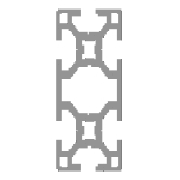
# Autodesk Inventor part: TRANSVERSAL (30X60)
Saved by Autodesk Inventor 2017 (Build 210142000, 142)
## iProperties
_CCFamilyDisplayName: 30-3060
_FrameMemberDoc: Frame Member File
_Version: 15.0.0
_GetPNFromCC: 1
Created: 2018-05-17
Part Number: TRANSVERSAL (30X60)
Material: Generic
Document SubType Name: Modeling
Standard: 8020 Metric
Designer: Luiz Gustavo
Manufacturer: 8020
Standards Organization: 8020 Metric
Language: en-US
Size Designation: 30-3060
Categories: <MemberInstance><Categories><Category DisplayName="Structural Shapes" InternalName="089c4875-fa83-4c05-b084-43b9cc11f5ed" Mnemonic="GRDR"><CategoryParameter DisplayName="Mass per Length Unit" InternalName="0bb95a10-148f-4027-a459-38d7b056702a" Mnemonic="shpmass"/><CategoryParameter DisplayName="Section Area" InternalName="1ff91680-64b0-4202-b9a3-7fd3f94bba3b" Mnemonic="secarea"/><CategoryParameter DisplayName="Radius of Gyration (x)" InternalName="25778675-03e9-40c1-b6a8-4a9ed693320d" Mnemonic="gyrradx"/><CategoryParameter DisplayName="Torsional Rigidity Modulus" InternalName="26c1ec35-5026-4c63-ad0a-751cf684a536" Mnemonic="torrigmod"/><CategoryParameter DisplayName="Distance of the Center of Gravity X-X" InternalName="26c9bdb8-9c79-4b4f-a92e-8e197583c9c4" Mnemonic="grcendistX"/><CategoryParameter DisplayName="Legacy Member ID" InternalName="340afe4f-75d7-48d3-ab7d-943f3c3da468" Mnemonic="LegacyMemberID"/><CategoryParameter DisplayName="Base Length" InternalName="42e34263-8f20-4d0e-ad48-bf1385b87c24" Mnemonic="shplen"/><CategoryParameter DisplayName="Moment of Inertia (y)" InternalName="4b9f58ea-bced-460e-81ea-3d29ca5a49e3" Mnemonic="inermomy"/><CategoryParameter DisplayName="Moment of Inertia (x)" InternalName="4cd780bc-73d7-43ac-917a-579e5cbd684d" Mnemonic="inermomx"/><CategoryParameter DisplayName="Custom Base Point" InternalName="4f1d1b73-316d-484b-a3df-9cbabb16eb77" Mnemonic="shpBasePoint"/><CategoryParameter DisplayName="Shape Height" InternalName="50274e7d-5ac0-4796-92cb-c59e54983c67" Mnemonic="shpheig"/><CategoryParameter DisplayName="Section Module (y)" InternalName="59eaa5e9-d227-48dc-b6c1-6920f96e0f95" Mnemonic="secmody"/><CategoryParameter DisplayName="Section Designation" InternalName="5a64d034-428d-49c8-ba32-7619764de20f" Mnemonic="shpdes"/><CategoryParameter DisplayName="Section Module (x)" InternalName="72cfad18-cf51-4ed4-aaa7-c6b224f8419f" Mnemonic="secmodx"/><CategoryParameter DisplayName="Torsional Section Modulus" InternalName="7c55a8dc-8844-49f9-a867-cc677b30ec9a" Mnemonic="torsecmod"/><CategoryParameter DisplayName="Shape Width" InternalName="7c717d54-a18f-4666-b4d4-573cce22c62c" Mnemonic="shpwdth"/><CategoryParameter DisplayName="Second Shape Thickness" InternalName="9251a8e1-85fd-4e47-af99-afdb762317d9" Mnemonic="shpthick2"/><CategoryParameter DisplayName="FG Authored" InternalName="9c666724-f362-4ea7-ac62-f6a007de5c69" Mnemonic="shpFGAuto"/><CategoryParameter DisplayName="Distance of the Center of Gravity Y-Y" InternalName="bcc4fb17-7af4-436a-8f8c-d0aa3b0248c5" Mnemonic="grcendistY"/><CategoryParameter DisplayName="Radius of Gyration (y)" InternalName="bfa18ebe-1636-4dbe-8d42-b263e0b73184" Mnemonic="gyrrady"/><CategoryParameter DisplayName="Shape Thickness" InternalName="d109cf76-8eb4-42fc-9800-4409734adc67" Mnemonic="shpthick"/><CategoryParameter DisplayName="Coefficient of Shear Displacement" InternalName="de4c90c6-aaa8-468f-a335-6737b311b5d3" Mnemonic="shdispc"/><Category DisplayName="Other" InternalName="f02205ff-2390-476f-921c-0b3185f88e84" Mnemonic="OTHSHP"><CategoryParameter DisplayName="Moment of Inertia (y)" InternalName="044c654e-f649-48ac-84cc-650a29ae31ca" Mnemonic="inermomy"/><CategoryParameter DisplayName="Shape Thickness" InternalName="12b1a788-9233-48fd-a933-2df8ff42b15f" Mnemonic="shpthick"/><CategoryParameter DisplayName="Mass per Length Unit" InternalName="2fd289d6-9394-4d2d-97e6-6659d7d4551d" Mnemonic="shpmass"/><CategoryParameter DisplayName="Radius of Gyration (y)" InternalName="743e1dfe-1bba-408b-b985-cf752b207386" Mnemonic="gyrrady"/><CategoryParameter DisplayName="Section Module (y)" InternalName="88b8bff9-a616-4028-93d5-ed4f79680d13" Mnemonic="secmody"/><CategoryParameter DisplayName="Section Area" InternalName="c46ecdf8-b6eb-4db9-8b25-30258930c1e3" Mnemonic="secarea"/><CategoryParameter DisplayName="Section Module (x)" InternalName="cac70804-9d39-43bb-be17-56ea1f39a6c2" Mnemonic="secmodx"/><CategoryParameter DisplayName="Moment of Inertia (x)" InternalName="ec6737bc-264f-43ed-b0bd-f6d410c2718d" Mnemonic="inermomx"/><CategoryParameter DisplayName="Radius of Gyration (x)" InternalName="ee72c61e-565e-4fd6-b448-66e1e1abcb7e" Mnemonic="gyrradx"/><Category DisplayName="8020" InternalName="79851eee-1260-43d5-80eb-d25638456875" Mnemonic="8020"/></Category></Category><Category DisplayName="DataType" InternalName="23b78d0f-2648-40c6-8793-ca6db495c9e8" Mnemonic="DATATYPE"><CategoryParameter DisplayName="DisplayName" InternalName="05415f3d-3907-474b-a020-eb9d644f4cf3" Mnemonic="DISPLAYNAME"/><CategoryParameter DisplayName="Standard" InternalName="0c0a119c-1e12-4c84-803f-101930972f5e" Mnemonic="STANDARD"/><CategoryParameter DisplayName="Description" InternalName="13903e3d-64b1-4950-80da-f627842ea37f" Mnemonic="DESCRIPTION"/><CategoryParameter DisplayName="Designation" InternalName="2675968c-4ce5-49e0-a4f5-552d29089031" Mnemonic="DESIGNATION"/><CategoryParameter DisplayName="Default Row" InternalName="2af9ec52-faaa-4026-b378-f9fa4afca842" Mnemonic="DEFAULTROW"/><CategoryParameter DisplayName="Folder Name" InternalName="3f06958e-8713-4116-9be7-ed6184ecc97b" Mnemonic="FOLDERNAME"/><CategoryParameter DisplayName="Revision Guid" InternalName="45a75005-10b1-4dfc-8d6d-dfe629f0b93c" Mnemonic="REVISIONGUID"/><CategoryParameter DisplayName="FileName" InternalName="8b46a4cc-9585-4fed-90c3-899f57e09a73" Mnemonic="FILENAME"/><CategoryParameter DisplayName="StdsOrg" InternalName="8f5914e1-4693-403f-8ab5-d37768198c9d" Mnemonic="STDSORG"/><CategoryParameter DisplayName="Family Version" InternalName="914462f6-6e19-4b14-ba84-155b9680b1d0" Mnemonic="FAMILYREVISION"/><CategoryParameter DisplayName="Standard Revision" InternalName="91d5a463-65c2-4fde-b823-3b7fea5e8e17" Mnemonic="STANDARDREVISION"/><CategoryParameter DisplayName="Member Revision" InternalName="a65d44b9-392f-4f4f-857b-e4b3d54996fe" Mnemonic="MEMBERREVISION"/><CategoryParameter DisplayName="ClipFormat" InternalName="bc51e27b-3422-4e78-93ef-cec197ddf230" Mnemonic="CLIPFORMAT"/><CategoryParameter DisplayName="Manufacturer" InternalName="cd6c7a72-a28a-4e50-99a9-2c7f4e13e5ad" Mnemonic="MANUFACTURER"/><CategoryParameter DisplayName="InternalName" InternalName="cf1d0246-76d9-4b4a-8305-fa0409afb5c1" Mnemonic="INTERNALNAME"/><CategoryParameter DisplayName="IsMetric" InternalName="e2385c5b-1ea4-4823-96a8-8de651266ec3" Mnemonic="ISMETRIC"/><Category DisplayName="Part" InternalName="c0e0b642-3bcb-4cc8-9e80-f96d35c4afa4" Mnemonic="PART"><CategoryParameter DisplayName="Part Number" InternalName="016b6077-bfbe-49bd-92c9-d8d59c39c941" Mnemonic="PARTNUMBER"/><CategoryParameter DisplayName="Stock Number" InternalName="4dba7c1c-e26c-444e-836c-b08b433409a8" Mnemonic="STOCKNUMBER"/><CategoryParameter DisplayName="Material Key" InternalName="5c9a8adb-dd2b-4535-b97f-0a94a95fe41f" Mnemonic="MATERIALKEY"/><CategoryParameter DisplayName="Material" InternalName="818a152a-d3c3-49ca-80ee-df7d91421b8e" Mnemonic="MATERIAL"/></Category></Category></Categories><FamilyTemplate Id="30-3060"><FamilyTemplateParameters><FamilyTemplateParameter ObjectType="kModelParameterObject" ValueType="xs:double" Id="12" ObjectReferenceKey="Length"/><FamilyTemplateParameter ObjectType="kPartComponentDefinitionObject" ValueType="xs:string" Id="23" SubObjectId="Material"/><FamilyTemplateParameter ObjectType="kPropertyObject" ValueType="xs:string" Id="26" ObjectReferenceKey="{32853F0F-3444-11d1-9E93-0060B03C1CA6}" SubObjectId="5"/><FamilyTemplateParameter ObjectType="kPropertyObject" ValueType="xs:string" Id="27" ObjectReferenceKey="{32853F0F-3444-11d1-9E93-0060B03C1CA6}" SubObjectId="52"/></FamilyTemplateParameters></FamilyTemplate><CategoryParameterMap><ParamToTemplateMap><ParamToTemplate CategoryParameter="//CategoryParameter[@InternalName='cf1d0246-76d9-4b4a-8305-fa0409afb5c1']" ConstantValue="ebd6c703-6585-4f80-969f-cab21f52a046"/><ParamToTemplate CategoryParameter="//CategoryParameter[@InternalName='45a75005-10b1-4dfc-8d6d-dfe629f0b93c']" ConstantValue="e073d83d-0598-4edb-9b1a-a79ba5c041d1"/><ParamToTemplate CategoryParameter="//CategoryParameter[@InternalName='3f06958e-8713-4116-9be7-ed6184ecc97b']" ConstantValue="30-3060"/><ParamToTemplate CategoryParameter="//CategoryParameter[@InternalName='8f5914e1-4693-403f-8ab5-d37768198c9d']" ConstantValue="8020 Metric"/><ParamToTemplate CategoryParameter="//CategoryParameter[@InternalName='0c0a119c-1e12-4c84-803f-101930972f5e']" TemplateParameter="18"/><ParamToTemplate CategoryParameter="//CategoryParameter[@InternalName='91d5a463-65c2-4fde-b823-3b7fea5e8e17']" TemplateParameter="19"/><ParamToTemplate CategoryParameter="//CategoryParameter[@InternalName='cd6c7a72-a28a-4e50-99a9-2c7f4e13e5ad']" ConstantValue="8020"/><ParamToTemplate CategoryParameter="//CategoryParameter[@InternalName='13903e3d-64b1-4950-80da-f627842ea37f']" TemplateParameter="22"/><ParamToTemplate CategoryParameter="//CategoryParameter[@InternalName='05415f3d-3907-474b-a020-eb9d644f4cf3']" ConstantValue="30-3060"/><ParamToTemplate CategoryParameter="//CategoryParameter[@InternalName='914462f6-6e19-4b14-ba84-155b9680b1d0']" ConstantValue="11"/><ParamToTemplate CategoryParameter="//CategoryParameter[@InternalName='bc51e27b-3422-4e78-93ef-cec197ddf230']" ConstantValue="CF_INVENTOR.STDPARTS"/><ParamToTemplate CategoryParameter="//CategoryParameter[@InternalName='e2385c5b-1ea4-4823-96a8-8de651266ec3']" ConstantValue="false"/><ParamToTemplate CategoryParameter="//CategoryParameter[@InternalName='2af9ec52-faaa-4026-b378-f9fa4afca842']" ConstantValue="1"/><ParamToTemplate CategoryParameter="//CategoryParameter[@InternalName='4f1d1b73-316d-484b-a3df-9cbabb16eb77']" ConstantValue="1"/><ParamToTemplate CategoryParameter="//CategoryParameter[@InternalName='9c666724-f362-4ea7-ac62-f6a007de5c69']" ConstantValue="1"/><ParamToTemplate CategoryParameter="//CategoryParameter[@InternalName='8b46a4cc-9585-4fed-90c3-899f57e09a73']" ConstantValue="30-3060"/><ParamToTemplate CategoryParameter="//CategoryParameter[@InternalName='a65d44b9-392f-4f4f-857b-e4b3d54996fe']" ConstantValue="3621f859-3cd7-4c8d-9d7e-184ee6a29b8c"/><ParamToTemplate CategoryParameter="//CategoryParameter[@InternalName='a65d44b9-392f-4f4f-857b-e4b3d54996fe']" ConstantValue="3621f859-3cd7-4c8d-9d7e-184ee6a29b8c"/><ParamToTemplate CategoryParameter="//CategoryParameter[@InternalName='2675968c-4ce5-49e0-a4f5-552d29089031']" TemplateParameter="27"/><ParamToTemplate CategoryParameter="//CategoryParameter[@InternalName='42e34263-8f20-4d0e-ad48-bf1385b87c24']" TemplateParameter="12"/><ParamToTemplate CategoryParameter="//CategoryParameter[@InternalName='818a152a-d3c3-49ca-80ee-df7d91421b8e']" TemplateParameter="23"/><ParamToTemplate CategoryParameter="//CategoryParameter[@InternalName='016b6077-bfbe-49bd-92c9-d8d59c39c941']" TemplateParameter="26"/></ParamToTemplateMap></CategoryParameterMap></MemberInstance>
Density: 1 g/cm^3
Appearance: Default
Mass: 87.8776 g
Surface Area: 850.531 cm^2
Volume: 87.8776 cm^3
IsCustomPart: 1
G_L: 150,0 mm
G_W: 30,000 mm
G_H: 60,000 mm
+2659EC03-3AEC-4DF6-9406-B24A7EDBFFC1+CUTDETAIL1: Cut
+68482761-B67A-421B-99FC-4A69EC554B32+CUTDETAIL2: Cut
Author: Luiz Gustavo
Autodesk Inventor part; units mm, degrees
sketch "30-3060" plane through (0, 0, 0) normal (0, 0, 1) x (1, 0, 0)
  arc A0 (20.03188, 67.433099) -> (20.41188, 67.0531) centre (20.41188, 67.433099) ccw
  line L0 (20.41188, 67.0531) -> (23.850873, 67.0531)
  arc A1 (23.850873, 67.0531) -> (24.231872, 67.434099) centre (23.850873, 67.434099) ccw
  line L1 (24.231872, 67.434099) -> (24.231872, 70.253094)
  arc A2 (24.231872, 70.253094) -> (23.231874, 71.253092) centre (23.231874, 70.253094) ccw
  line L2 (23.231874, 71.253092) -> (20.41288, 71.253092)
  arc A3 (20.41288, 71.253092) -> (20.03188, 70.872092) centre (20.41288, 70.872092) ccw
  line L3 (20.03188, 70.872092) -> (20.03188, 67.433099)
  arc A4 (14.356985, 59.871616) -> (12.850396, 61.378204) centre (13.519276, 60.540496) ccw
  line L4 (12.850396, 61.378204) -> (11.871278, 60.596414)
  arc A5 (11.871278, 60.596414) -> (9.18326, 60.592322) centre (10.531899, 57.553119) ccw
  line L5 (9.18326, 60.592322) -> (8.204141, 61.374112)
  arc A6 (8.204141, 61.374112) -> (6.697553, 59.867523) centre (7.535262, 60.536403) ccw
  line L6 (6.697553, 59.867523) -> (7.484165, 58.882365)
  arc A7 (7.484165, 58.882365) -> (7.488604, 56.213741) centre (10.531899, 57.553119) ccw
  line L7 (7.488604, 56.213741) -> (6.706814, 55.234622)
  arc A8 (6.706814, 55.234622) -> (8.213402, 53.728034) centre (7.544523, 54.565743) ccw
  line L8 (8.213402, 53.728034) -> (9.192521, 54.509824)
  arc A9 (9.192521, 54.509824) -> (11.871278, 54.509824) centre (10.531899, 57.553119) ccw
  line L9 (11.871278, 54.509824) -> (12.850396, 53.728034)
  arc A10 (12.850396, 53.728034) -> (14.356985, 55.234622) centre (13.519276, 54.565743) ccw
  line L10 (14.356985, 55.234622) -> (13.575195, 56.213741)
  arc A11 (13.575195, 56.213741) -> (13.575195, 58.892497) centre (10.531899, 57.553119) ccw
  line L11 (13.575195, 58.892497) -> (14.356985, 59.871616)
  arc A12 (14.356985, 29.871676) -> (12.850396, 31.378264) centre (13.519276, 30.540556) ccw
  line L12 (12.850396, 31.378264) -> (11.871278, 30.596474)
  arc A13 (11.871278, 30.596474) -> (9.18326, 30.592382) centre (10.531899, 27.553179) ccw
  line L13 (9.18326, 30.592382) -> (8.204141, 31.374172)
  arc A14 (8.204141, 31.374172) -> (6.697553, 29.867583) centre (7.535262, 30.536463) ccw
  line L14 (6.697553, 29.867583) -> (7.484165, 28.882425)
  arc A15 (7.484165, 28.882425) -> (7.488604, 26.213801) centre (10.531899, 27.553179) ccw
  line L15 (7.488604, 26.213801) -> (6.706814, 25.234682)
  arc A16 (6.706814, 25.234682) -> (8.213402, 23.728094) centre (7.544523, 24.565803) ccw
  line L16 (8.213402, 23.728094) -> (9.192521, 24.509884)
  arc A17 (9.192521, 24.509884) -> (11.871278, 24.509884) centre (10.531899, 27.553179) ccw
  line L17 (11.871278, 24.509884) -> (12.850396, 23.728094)
  arc A18 (12.850396, 23.728094) -> (14.356985, 25.234682) centre (13.519276, 24.565803) ccw
  line L18 (14.356985, 25.234682) -> (13.575195, 26.213801)
  arc A19 (13.575195, 26.213801) -> (13.575195, 28.892557) centre (10.531899, 27.553179) ccw
  line L19 (13.575195, 28.892557) -> (14.356985, 29.871676)
  arc A20 (23.231874, 13.853206) -> (24.231872, 14.853204) centre (23.231874, 14.853204) ccw
  line L20 (24.231872, 14.853204) -> (24.231872, 17.672199)
  arc A21 (24.231872, 17.672199) -> (23.850873, 18.053198) centre (23.850873, 17.672199) ccw
  line L21 (23.850873, 18.053198) -> (20.41188, 18.053198)
  arc A22 (20.41188, 18.053198) -> (20.03188, 17.673199) centre (20.41188, 17.673199) ccw
  line L22 (20.03188, 17.673199) -> (20.03188, 14.234206)
  arc A23 (20.03188, 14.234206) -> (20.41288, 13.853206) centre (20.41288, 14.234206) ccw
  line L23 (20.41288, 13.853206) -> (23.231874, 13.853206)
  line L24 (-2.210601, 49.820584) -> (-2.210601, 52.990619)
  arc A24 (-2.210601, 49.820584) -> (-1.710906, 49.303136) centre (-1.710906, 49.803135) ccw
  line L25 (0.271691, 49.303136) -> (-1.710906, 49.303136)
  arc A25 (0.271691, 49.303136) -> (0.625243, 49.449582) centre (0.271691, 49.803135) ccw
  line L26 (4.55077, 53.375108) -> (0.625243, 49.449582)
  arc A26 (4.55077, 53.375108) -> (4.697216, 53.728661) centre (4.197217, 53.728661) ccw
  line L27 (4.697216, 56.603121) -> (4.697216, 53.728661)
  line L28 (5.207215, 57.553119) -> (4.697216, 56.603121)
  line L29 (4.697216, 58.503117) -> (5.207215, 57.553119)
  line L30 (4.697216, 61.377577) -> (4.697216, 58.503117)
  arc A27 (4.697216, 61.377577) -> (4.55077, 61.73113) centre (4.197217, 61.377577) ccw
  line L31 (0.625243, 65.656656) -> (4.55077, 61.73113)
  arc A28 (0.625243, 65.656656) -> (0.271691, 65.803103) centre (0.271691, 65.303104) ccw
  line L32 (-1.710906, 65.803103) -> (0.271691, 65.803103)
  arc A29 (-1.710906, 65.803103) -> (-2.210601, 65.285654) centre (-1.710906, 65.303104) ccw
  line L33 (-2.210601, 61.990619) -> (-2.210601, 65.285654)
  arc A30 (-2.710601, 61.490619) -> (-2.210601, 61.990619) centre (-2.710601, 61.990619) ccw
  line L34 (-3.968071, 61.490619) -> (-2.710601, 61.490619)
  arc A31 (-4.468071, 61.990619) -> (-3.968071, 61.490619) centre (-3.968071, 61.990619) ccw
  line L35 (-4.468071, 70.553093) -> (-4.468071, 61.990619)
  arc A32 (-2.468075, 72.553089) -> (-4.468071, 70.553093) centre (-2.468075, 70.553093) ccw
  line L36 (5.969399, 72.553089) -> (-2.468075, 72.553089)
  arc A33 (6.469399, 72.053089) -> (5.969399, 72.553089) centre (5.969399, 72.053089) ccw
  line L37 (6.469399, 70.795619) -> (6.469399, 72.053089)
  arc A34 (5.969399, 70.295619) -> (6.469399, 70.795619) centre (5.969399, 70.795619) ccw
  line L38 (2.799364, 70.295619) -> (5.969399, 70.295619)
  arc A35 (2.799364, 70.295619) -> (2.281916, 69.795925) centre (2.781915, 69.795925) ccw
  line L39 (2.281916, 67.813328) -> (2.281916, 69.795925)
  arc A36 (2.281916, 67.813328) -> (2.428362, 67.459775) centre (2.781915, 67.813328) ccw
  line L40 (6.353888, 63.534249) -> (2.428362, 67.459775)
  arc A37 (6.353888, 63.534249) -> (6.707441, 63.387802) centre (6.707441, 63.887801) ccw
  line L41 (9.519401, 63.387802) -> (6.707441, 63.387802)
  line L42 (10.469399, 62.877803) -> (9.519401, 63.387802)
  line L43 (11.419397, 63.387802) -> (10.469399, 62.877803)
  line L44 (14.356358, 63.387802) -> (11.419397, 63.387802)
  arc A38 (14.356358, 63.387802) -> (14.70991, 63.534249) centre (14.356358, 63.887801) ccw
  line L45 (18.635436, 67.459775) -> (14.70991, 63.534249)
  arc A39 (18.635436, 67.459775) -> (18.781883, 67.813328) centre (18.281884, 67.813328) ccw
  line L46 (18.781883, 69.795925) -> (18.781883, 67.813328)
  arc A40 (18.781883, 69.795925) -> (18.264434, 70.295619) centre (18.281884, 69.795925) ccw
  line L47 (14.969399, 70.295619) -> (18.264434, 70.295619)
  arc A41 (14.469399, 70.795619) -> (14.969399, 70.295619) centre (14.969399, 70.795619) ccw
  line L48 (14.469399, 72.053089) -> (14.469399, 70.795619)
  arc A42 (14.969399, 72.553089) -> (14.469399, 72.053089) centre (14.969399, 72.053089) ccw
  line L49 (23.531873, 72.553089) -> (14.969399, 72.553089)
  arc A43 (25.531869, 70.553093) -> (23.531873, 72.553089) centre (23.531873, 70.553093) ccw
  line L50 (25.531869, 62.115619) -> (25.531869, 70.553093)
  arc A44 (25.031869, 61.615619) -> (25.531869, 62.115619) centre (25.031869, 62.115619) ccw
  line L51 (23.774399, 61.615619) -> (25.031869, 61.615619)
  arc A45 (23.274399, 62.115619) -> (23.774399, 61.615619) centre (23.774399, 62.115619) ccw
  line L52 (23.274399, 65.285654) -> (23.274399, 62.115619)
  arc A46 (23.274399, 65.285654) -> (22.774705, 65.803103) centre (22.774705, 65.303104) ccw
  line L53 (20.792108, 65.803103) -> (22.774705, 65.803103)
  arc A47 (20.792108, 65.803103) -> (20.438555, 65.656656) centre (20.792108, 65.303104) ccw
  line L54 (16.513029, 61.73113) -> (20.438555, 65.656656)
  arc A48 (16.513029, 61.73113) -> (16.366583, 61.377577) centre (16.866582, 61.377577) ccw
  line L55 (16.366583, 58.503117) -> (16.366583, 61.377577)
  line L56 (15.856584, 57.553119) -> (16.366583, 58.503117)
  line L57 (16.366583, 56.603121) -> (15.856584, 57.553119)
  line L58 (16.366583, 53.728661) -> (16.366583, 56.603121)
  arc A49 (16.366583, 53.728661) -> (16.513029, 53.375108) centre (16.866582, 53.728661) ccw
  line L59 (20.438555, 49.449582) -> (16.513029, 53.375108)
  arc A50 (20.438555, 49.449582) -> (20.792108, 49.303136) centre (20.792108, 49.803135) ccw
  line L60 (22.774705, 49.303136) -> (20.792108, 49.303136)
  arc A51 (22.774705, 49.303136) -> (23.274399, 49.820584) centre (22.774705, 49.803135) ccw
  line L61 (23.274399, 53.115619) -> (23.274399, 49.820584)
  arc A52 (23.774399, 53.615619) -> (23.274399, 53.115619) centre (23.774399, 53.115619) ccw
  line L62 (25.031869, 53.615619) -> (23.774399, 53.615619)
  arc A53 (25.531869, 53.115619) -> (25.031869, 53.615619) centre (25.031869, 53.115619) ccw
  line L63 (25.531869, 31.990679) -> (25.531869, 53.115619)
  arc A54 (25.031869, 31.490679) -> (25.531869, 31.990679) centre (25.031869, 31.990679) ccw
  line L64 (23.774399, 31.490679) -> (25.031869, 31.490679)
  arc A55 (23.274399, 31.990679) -> (23.774399, 31.490679) centre (23.774399, 31.990679) ccw
  line L65 (23.274399, 35.285714) -> (23.274399, 31.990679)
  arc A56 (23.274399, 35.285714) -> (22.774705, 35.803163) centre (22.774705, 35.303164) ccw
  line L66 (20.792108, 35.803163) -> (22.774705, 35.803163)
  arc A57 (20.792108, 35.803163) -> (20.438555, 35.656716) centre (20.792108, 35.303164) ccw
  line L67 (16.513029, 31.73119) -> (20.438555, 35.656716)
  arc A58 (16.513029, 31.73119) -> (16.366583, 31.377637) centre (16.866582, 31.377637) ccw
  line L68 (16.366583, 28.503177) -> (16.366583, 31.377637)
  line L69 (15.856584, 27.553179) -> (16.366583, 28.503177)
  line L70 (16.366583, 26.603181) -> (15.856584, 27.553179)
  line L71 (16.366583, 23.728721) -> (16.366583, 26.603181)
  arc A59 (16.366583, 23.728721) -> (16.513029, 23.375168) centre (16.866582, 23.728721) ccw
  line L72 (20.438555, 19.449642) -> (16.513029, 23.375168)
  arc A60 (20.438555, 19.449642) -> (20.792108, 19.303196) centre (20.792108, 19.803195) ccw
  line L73 (22.774705, 19.303196) -> (20.792108, 19.303196)
  arc A61 (22.774705, 19.303196) -> (23.274399, 19.820644) centre (22.774705, 19.803195) ccw
  line L74 (23.274399, 22.990679) -> (23.274399, 19.820644)
  arc A62 (23.774399, 23.490679) -> (23.274399, 22.990679) centre (23.774399, 22.990679) ccw
  line L75 (25.031869, 23.490679) -> (23.774399, 23.490679)
  arc A63 (25.531869, 22.990679) -> (25.031869, 23.490679) centre (25.031869, 22.990679) ccw
  line L76 (25.531869, 14.553205) -> (25.531869, 22.990679)
  arc A64 (23.531873, 12.553209) -> (25.531869, 14.553205) centre (23.531873, 14.553205) ccw
  line L77 (14.969399, 12.553209) -> (23.531873, 12.553209)
  arc A65 (14.469399, 13.053209) -> (14.969399, 12.553209) centre (14.969399, 13.053209) ccw
  line L78 (14.469399, 14.310679) -> (14.469399, 13.053209)
  arc A66 (14.969399, 14.810679) -> (14.469399, 14.310679) centre (14.969399, 14.310679) ccw
  line L79 (18.264434, 14.810679) -> (14.969399, 14.810679)
  arc A67 (18.264434, 14.810679) -> (18.781883, 15.310373) centre (18.281884, 15.310373) ccw
  line L80 (18.781883, 17.292971) -> (18.781883, 15.310373)
  arc A68 (18.781883, 17.292971) -> (18.635436, 17.646523) centre (18.281884, 17.292971) ccw
  line L81 (14.70991, 21.572049) -> (18.635436, 17.646523)
  arc A69 (14.70991, 21.572049) -> (14.356358, 21.718496) centre (14.356358, 21.218497) ccw
  line L82 (11.419397, 21.718496) -> (14.356358, 21.718496)
  line L83 (10.469399, 22.228495) -> (11.419397, 21.718496)
  line L84 (9.519401, 21.718496) -> (10.469399, 22.228495)
  line L85 (6.707441, 21.718496) -> (9.519401, 21.718496)
  arc A70 (6.707441, 21.718496) -> (6.353888, 21.572049) centre (6.707441, 21.218497) ccw
  line L86 (2.428362, 17.646523) -> (6.353888, 21.572049)
  arc A71 (2.428362, 17.646523) -> (2.281916, 17.292971) centre (2.781915, 17.292971) ccw
  line L87 (2.281916, 15.310373) -> (2.281916, 17.292971)
  arc A72 (2.281916, 15.310373) -> (2.799364, 14.810679) centre (2.781915, 15.310373) ccw
  line L88 (5.969399, 14.810679) -> (2.799364, 14.810679)
  arc A73 (6.469399, 14.310679) -> (5.969399, 14.810679) centre (5.969399, 14.310679) ccw
  line L89 (6.469399, 13.053209) -> (6.469399, 14.310679)
  arc A74 (5.969399, 12.553209) -> (6.469399, 13.053209) centre (5.969399, 13.053209) ccw
  line L90 (-2.468075, 12.553209) -> (5.969399, 12.553209)
  arc A75 (-4.468071, 14.553205) -> (-2.468075, 12.553209) centre (-2.468075, 14.553205) ccw
  line L91 (-4.468071, 23.115679) -> (-4.468071, 14.553205)
  arc A76 (-3.968071, 23.615679) -> (-4.468071, 23.115679) centre (-3.968071, 23.115679) ccw
  line L92 (-2.710601, 23.615679) -> (-3.968071, 23.615679)
  arc A77 (-2.210601, 23.115679) -> (-2.710601, 23.615679) centre (-2.710601, 23.115679) ccw
  line L93 (-2.210601, 19.820644) -> (-2.210601, 23.115679)
  arc A78 (-2.210601, 19.820644) -> (-1.710906, 19.303196) centre (-1.710906, 19.803195) ccw
  line L94 (0.271691, 19.303196) -> (-1.710906, 19.303196)
  arc A79 (0.271691, 19.303196) -> (0.625243, 19.449642) centre (0.271691, 19.803195) ccw
  line L95 (4.55077, 23.375168) -> (0.625243, 19.449642)
  arc A80 (4.55077, 23.375168) -> (4.697216, 23.728721) centre (4.197217, 23.728721) ccw
  line L96 (4.697216, 26.603181) -> (4.697216, 23.728721)
  line L97 (5.207215, 27.553179) -> (4.697216, 26.603181)
  line L98 (4.697216, 28.503177) -> (5.207215, 27.553179)
  line L99 (4.697216, 31.377637) -> (4.697216, 28.503177)
  arc A81 (4.697216, 31.377637) -> (4.55077, 31.73119) centre (4.197217, 31.377637) ccw
  line L100 (0.625243, 35.656716) -> (4.55077, 31.73119)
  arc A82 (0.625243, 35.656716) -> (0.271691, 35.803163) centre (0.271691, 35.303164) ccw
  line L101 (-1.710906, 35.803163) -> (0.271691, 35.803163)
  arc A83 (-1.710906, 35.803163) -> (-2.210601, 35.285714) centre (-1.710906, 35.303164) ccw
  line L102 (-2.210601, 32.115679) -> (-2.210601, 35.285714)
  arc A84 (-2.710601, 31.615679) -> (-2.210601, 32.115679) centre (-2.710601, 32.115679) ccw
  line L103 (-3.968071, 31.615679) -> (-2.710601, 31.615679)
  arc A85 (-4.468071, 32.115679) -> (-3.968071, 31.615679) centre (-3.968071, 32.115679) ccw
  line L104 (-4.468071, 52.990619) -> (-4.468071, 32.115679)
  arc A86 (-3.968071, 53.490619) -> (-4.468071, 52.990619) centre (-3.968071, 52.990619) ccw
  line L105 (-2.710601, 53.490619) -> (-3.968071, 53.490619)
  arc A87 (-2.210601, 52.990619) -> (-2.710601, 53.490619) centre (-2.710601, 52.990619) ccw
  arc A88 (1.031918, 17.673199) -> (0.651919, 18.053198) centre (0.651919, 17.673199) ccw
  line L106 (0.651919, 18.053198) -> (-2.787074, 18.053198)
  arc A89 (-2.787074, 18.053198) -> (-3.168073, 17.672199) centre (-2.787074, 17.672199) ccw
  line L107 (-3.168073, 17.672199) -> (-3.168073, 14.853204)
  arc A90 (-3.168073, 14.853204) -> (-2.168075, 13.853206) centre (-2.168075, 14.853204) ccw
  line L108 (-2.168075, 13.853206) -> (0.650919, 13.853206)
  arc A91 (0.650919, 13.853206) -> (1.031918, 14.234206) centre (0.650919, 14.234206) ccw
  line L109 (1.031918, 14.234206) -> (1.031918, 17.673199)
  arc A92 (23.331874, 46.603141) -> (22.831875, 47.10314) centre (22.831875, 46.603141) ccw
  line L110 (22.831875, 47.10314) -> (19.800079, 47.10314)
  arc A93 (18.739421, 47.542479) -> (19.800079, 47.10314) centre (19.800079, 48.603137) ccw
  line L111 (18.739421, 47.542479) -> (14.70991, 51.571989)
  arc A94 (14.70991, 51.571989) -> (14.356358, 51.718436) centre (14.356358, 51.218437) ccw
  line L112 (14.356358, 51.718436) -> (11.419397, 51.718436)
  line L113 (11.419397, 51.718436) -> (10.469399, 52.228435)
  line L114 (10.469399, 52.228435) -> (9.519401, 51.718436)
  line L115 (9.519401, 51.718436) -> (6.707441, 51.718436)
  arc A95 (6.707441, 51.718436) -> (6.353888, 51.571989) centre (6.707441, 51.218437) ccw
  line L116 (6.353888, 51.571989) -> (2.324378, 47.542479)
  arc A96 (1.26372, 47.10314) -> (2.324378, 47.542479) centre (1.26372, 48.603137) ccw
  line L117 (1.26372, 47.10314) -> (-1.768076, 47.10314)
  arc A97 (-1.768076, 47.10314) -> (-2.268075, 46.603141) centre (-1.768076, 46.603141) ccw
  line L118 (-2.268075, 46.603141) -> (-2.268075, 38.503157)
  arc A98 (-2.268075, 38.503157) -> (-1.768076, 38.003158) centre (-1.768076, 38.503157) ccw
  line L119 (-1.768076, 38.003158) -> (1.26372, 38.003158)
  arc A99 (2.324378, 37.563819) -> (1.26372, 38.003158) centre (1.26372, 36.503161) ccw
  line L120 (2.324378, 37.563819) -> (6.353888, 33.534309)
  arc A100 (6.353888, 33.534309) -> (6.707441, 33.387862) centre (6.707441, 33.887861) ccw
  line L121 (6.707441, 33.387862) -> (9.519401, 33.387862)
  line L122 (9.519401, 33.387862) -> (10.469399, 32.877863)
  line L123 (10.469399, 32.877863) -> (11.419397, 33.387862)
  line L124 (11.419397, 33.387862) -> (14.356358, 33.387862)
  arc A101 (14.356358, 33.387862) -> (14.70991, 33.534309) centre (14.356358, 33.887861) ccw
  line L125 (14.70991, 33.534309) -> (18.739421, 37.563819)
  arc A102 (19.800079, 38.003158) -> (18.739421, 37.563819) centre (19.800079, 36.503161) ccw
  line L126 (19.800079, 38.003158) -> (22.831875, 38.003158)
  arc A103 (22.831875, 38.003158) -> (23.331874, 38.503157) centre (22.831875, 38.503157) ccw
  line L127 (23.331874, 38.503157) -> (23.331874, 46.603141)
  arc A104 (0.651919, 67.0531) -> (1.031918, 67.433099) centre (0.651919, 67.433099) ccw
  line L128 (1.031918, 67.433099) -> (1.031918, 70.872092)
  arc A105 (1.031918, 70.872092) -> (0.650919, 71.253092) centre (0.650919, 70.872092) ccw
  line L129 (0.650919, 71.253092) -> (-2.168075, 71.253092)
  arc A106 (-2.168075, 71.253092) -> (-3.168073, 70.253094) centre (-2.168075, 70.253094) ccw
  line L130 (-3.168073, 70.253094) -> (-3.168073, 67.434099)
  arc A107 (-3.168073, 67.434099) -> (-2.787074, 67.0531) centre (-2.787074, 67.434099) ccw
  line L131 (-2.787074, 67.0531) -> (0.651919, 67.0531)
ref_plane "Start Plane" through (0, 0, -22.007503) normal (0, 0, 1) x (1, 0, 0)
ref_plane "End Plane" through (0, 0, 128.000817) normal (0, 0, 1) x (1, 0, 0)
sketch "Sketch" plane through (0, 0, 0) normal (0, 0, 1) x (1, 0, 0)
  arc A0 (9.499981, 39.87992) -> (9.87998, 39.499921) centre (9.87998, 39.87992) ccw
  line L0 (9.87998, 39.499921) -> (13.318973, 39.499921)
  arc A1 (13.318973, 39.499921) -> (13.699973, 39.88092) centre (13.318973, 39.88092) ccw
  line L1 (13.699973, 39.88092) -> (13.699973, 42.699915)
  arc A2 (13.699973, 42.699915) -> (12.699975, 43.699913) centre (12.699975, 42.699915) ccw
  line L2 (12.699975, 43.699913) -> (9.88098, 43.699913)
  arc A3 (9.88098, 43.699913) -> (9.499981, 43.318913) centre (9.88098, 43.318913) ccw
  line L3 (9.499981, 43.318913) -> (9.499981, 39.87992)
  arc A4 (3.825085, 32.318437) -> (2.318497, 33.825025) centre (2.987376, 32.987316) ccw
  line L4 (2.318497, 33.825025) -> (1.339378, 33.043235)
  arc A5 (1.339378, 33.043235) -> (-1.34864, 33.039143) centre (0, 29.99994) ccw
  line L5 (-1.34864, 33.039143) -> (-2.327758, 33.820933)
  arc A6 (-2.327758, 33.820933) -> (-3.834347, 32.314344) centre (-2.996638, 32.983224) ccw
  line L6 (-3.834347, 32.314344) -> (-3.047734, 31.329186)
  arc A7 (-3.047734, 31.329186) -> (-3.043295, 28.660562) centre (0, 29.99994) ccw
  line L7 (-3.043295, 28.660562) -> (-3.825085, 27.681443)
  arc A8 (-3.825085, 27.681443) -> (-2.318497, 26.174855) centre (-2.987376, 27.012564) ccw
  line L8 (-2.318497, 26.174855) -> (-1.339378, 26.956645)
  arc A9 (-1.339378, 26.956645) -> (1.339378, 26.956645) centre (0, 29.99994) ccw
  line L9 (1.339378, 26.956645) -> (2.318497, 26.174855)
  arc A10 (2.318497, 26.174855) -> (3.825085, 27.681443) centre (2.987376, 27.012564) ccw
  line L10 (3.825085, 27.681443) -> (3.043295, 28.660562)
  arc A11 (3.043295, 28.660562) -> (3.043295, 31.339318) centre (0, 29.99994) ccw
  line L11 (3.043295, 31.339318) -> (3.825085, 32.318437)
  arc A12 (3.825085, 2.318497) -> (2.318497, 3.825085) centre (2.987376, 2.987376) ccw
  line L12 (2.318497, 3.825085) -> (1.339378, 3.043295)
  arc A13 (1.339378, 3.043295) -> (-1.34864, 3.039203) centre (0, 0) ccw
  line L13 (-1.34864, 3.039203) -> (-2.327758, 3.820993)
  arc A14 (-2.327758, 3.820993) -> (-3.834347, 2.314404) centre (-2.996638, 2.983284) ccw
  line L14 (-3.834347, 2.314404) -> (-3.047734, 1.329246)
  arc A15 (-3.047734, 1.329246) -> (-3.043295, -1.339378) centre (0, 0) ccw
  line L15 (-3.043295, -1.339378) -> (-3.825085, -2.318497)
  arc A16 (-3.825085, -2.318497) -> (-2.318497, -3.825085) centre (-2.987376, -2.987376) ccw
  line L16 (-2.318497, -3.825085) -> (-1.339378, -3.043295)
  arc A17 (-1.339378, -3.043295) -> (1.339378, -3.043295) centre (0, 0) ccw
  line L17 (1.339378, -3.043295) -> (2.318497, -3.825085)
  arc A18 (2.318497, -3.825085) -> (3.825085, -2.318497) centre (2.987376, -2.987376) ccw
  line L18 (3.825085, -2.318497) -> (3.043295, -1.339378)
  arc A19 (3.043295, -1.339378) -> (3.043295, 1.339378) centre (0, 0) ccw
  line L19 (3.043295, 1.339378) -> (3.825085, 2.318497)
  arc A20 (12.699975, -13.699973) -> (13.699973, -12.699975) centre (12.699975, -12.699975) ccw
  line L20 (13.699973, -12.699975) -> (13.699973, -9.88098)
  arc A21 (13.699973, -9.88098) -> (13.318973, -9.499981) centre (13.318973, -9.88098) ccw
  line L21 (13.318973, -9.499981) -> (9.87998, -9.499981)
  arc A22 (9.87998, -9.499981) -> (9.499981, -9.87998) centre (9.87998, -9.87998) ccw
  line L22 (9.499981, -9.87998) -> (9.499981, -13.318973)
  arc A23 (9.499981, -13.318973) -> (9.88098, -13.699973) centre (9.88098, -13.318973) ccw
  line L23 (9.88098, -13.699973) -> (12.699975, -13.699973)
  line L24 (-12.7425, 22.267405) -> (-12.7425, 25.43744)
  arc A24 (-12.7425, 22.267405) -> (-12.242806, 21.749957) centre (-12.242806, 22.249955) ccw
  line L25 (-10.260209, 21.749956) -> (-12.242806, 21.749957)
  arc A25 (-10.260209, 21.749956) -> (-9.906656, 21.896403) centre (-10.260209, 22.249955) ccw
  line L26 (-5.98113, 25.821929) -> (-9.906656, 21.896403)
  arc A26 (-5.98113, 25.821929) -> (-5.834683, 26.175482) centre (-6.334682, 26.175482) ccw
  line L27 (-5.834683, 29.049942) -> (-5.834683, 26.175482)
  line L28 (-5.324684, 29.99994) -> (-5.834683, 29.049942)
  line L29 (-5.834683, 30.949938) -> (-5.324684, 29.99994)
  line L30 (-5.834683, 33.824398) -> (-5.834683, 30.949938)
  arc A27 (-5.834683, 33.824398) -> (-5.98113, 34.177951) centre (-6.334682, 33.824398) ccw
  line L31 (-9.906656, 38.103477) -> (-5.98113, 34.177951)
  arc A28 (-9.906656, 38.103477) -> (-10.260209, 38.249923) centre (-10.260209, 37.749925) ccw
  line L32 (-12.242806, 38.249924) -> (-10.260209, 38.249923)
  arc A29 (-12.242806, 38.249924) -> (-12.7425, 37.732475) centre (-12.242806, 37.749924) ccw
  line L33 (-12.7425, 34.43744) -> (-12.7425, 37.732475)
  arc A30 (-13.2425, 33.93744) -> (-12.7425, 34.43744) centre (-13.2425, 34.43744) ccw
  line L34 (-14.49997, 33.93744) -> (-13.2425, 33.93744)
  arc A31 (-14.99997, 34.43744) -> (-14.49997, 33.93744) centre (-14.49997, 34.43744) ccw
  line L35 (-14.99997, 42.999914) -> (-14.99997, 34.43744)
  arc A32 (-12.999974, 44.99991) -> (-14.99997, 42.999914) centre (-12.999974, 42.999914) ccw
  line L36 (-4.5625, 44.99991) -> (-12.999974, 44.99991)
  arc A33 (-4.0625, 44.49991) -> (-4.5625, 44.99991) centre (-4.5625, 44.49991) ccw
  line L37 (-4.0625, 43.24244) -> (-4.0625, 44.49991)
  arc A34 (-4.5625, 42.74244) -> (-4.0625, 43.24244) centre (-4.5625, 43.24244) ccw
  line L38 (-7.732535, 42.74244) -> (-4.5625, 42.74244)
  arc A35 (-7.732535, 42.74244) -> (-8.249983, 42.242746) centre (-7.749985, 42.242746) ccw
  line L39 (-8.249984, 40.260149) -> (-8.249983, 42.242746)
  arc A36 (-8.249984, 40.260149) -> (-8.103537, 39.906596) centre (-7.749985, 40.260149) ccw
  line L40 (-4.178011, 35.98107) -> (-8.103537, 39.906596)
  arc A37 (-4.178011, 35.98107) -> (-3.824458, 35.834623) centre (-3.824458, 36.334622) ccw
  line L41 (-1.012498, 35.834623) -> (-3.824458, 35.834623)
  line L42 (-0.0625, 35.324624) -> (-1.012498, 35.834623)
  line L43 (0.887498, 35.834623) -> (-0.0625, 35.324624)
  line L44 (3.824458, 35.834623) -> (0.887498, 35.834623)
  arc A38 (3.824458, 35.834623) -> (4.178011, 35.98107) centre (3.824458, 36.334622) ccw
  line L45 (8.103537, 39.906596) -> (4.178011, 35.98107)
  arc A39 (8.103537, 39.906596) -> (8.249983, 40.260149) centre (7.749985, 40.260149) ccw
  line L46 (8.249984, 42.242746) -> (8.249983, 40.260149)
  arc A40 (8.249984, 42.242746) -> (7.732535, 42.74244) centre (7.749984, 42.242746) ccw
  line L47 (4.4375, 42.74244) -> (7.732535, 42.74244)
  arc A41 (3.9375, 43.24244) -> (4.4375, 42.74244) centre (4.4375, 43.24244) ccw
  line L48 (3.9375, 44.49991) -> (3.9375, 43.24244)
  arc A42 (4.4375, 44.99991) -> (3.9375, 44.49991) centre (4.4375, 44.49991) ccw
  line L49 (12.999974, 44.99991) -> (4.4375, 44.99991)
  arc A43 (14.99997, 42.999914) -> (12.999974, 44.99991) centre (12.999974, 42.999914) ccw
  line L50 (14.99997, 34.56244) -> (14.99997, 42.999914)
  arc A44 (14.49997, 34.06244) -> (14.99997, 34.56244) centre (14.49997, 34.56244) ccw
  line L51 (13.2425, 34.06244) -> (14.49997, 34.06244)
  arc A45 (12.7425, 34.56244) -> (13.2425, 34.06244) centre (13.2425, 34.56244) ccw
  line L52 (12.7425, 37.732475) -> (12.7425, 34.56244)
  arc A46 (12.7425, 37.732475) -> (12.242806, 38.249923) centre (12.242806, 37.749925) ccw
  line L53 (10.260209, 38.249924) -> (12.242806, 38.249923)
  arc A47 (10.260209, 38.249924) -> (9.906656, 38.103477) centre (10.260209, 37.749924) ccw
  line L54 (5.98113, 34.177951) -> (9.906656, 38.103477)
  arc A48 (5.98113, 34.177951) -> (5.834683, 33.824398) centre (6.334682, 33.824398) ccw
  line L55 (5.834683, 30.949938) -> (5.834683, 33.824398)
  line L56 (5.324684, 29.99994) -> (5.834683, 30.949938)
  line L57 (5.834683, 29.049942) -> (5.324684, 29.99994)
  line L58 (5.834683, 26.175482) -> (5.834683, 29.049942)
  arc A49 (5.834683, 26.175482) -> (5.98113, 25.821929) centre (6.334682, 26.175482) ccw
  line L59 (9.906656, 21.896403) -> (5.98113, 25.821929)
  arc A50 (9.906656, 21.896403) -> (10.260209, 21.749957) centre (10.260209, 22.249955) ccw
  line L60 (12.242806, 21.749956) -> (10.260209, 21.749957)
  arc A51 (12.242806, 21.749956) -> (12.7425, 22.267405) centre (12.242806, 22.249955) ccw
  line L61 (12.7425, 25.56244) -> (12.7425, 22.267405)
  arc A52 (13.2425, 26.06244) -> (12.7425, 25.56244) centre (13.2425, 25.56244) ccw
  line L62 (14.49997, 26.06244) -> (13.2425, 26.06244)
  arc A53 (14.99997, 25.56244) -> (14.49997, 26.06244) centre (14.49997, 25.56244) ccw
  line L63 (14.99997, 4.4375) -> (14.99997, 25.56244)
  arc A54 (14.49997, 3.9375) -> (14.99997, 4.4375) centre (14.49997, 4.4375) ccw
  line L64 (13.2425, 3.9375) -> (14.49997, 3.9375)
  arc A55 (12.7425, 4.4375) -> (13.2425, 3.9375) centre (13.2425, 4.4375) ccw
  line L65 (12.7425, 7.732535) -> (12.7425, 4.4375)
  arc A56 (12.7425, 7.732535) -> (12.242806, 8.249984) centre (12.242806, 7.749984) ccw
  line L66 (10.260209, 8.249983) -> (12.242806, 8.249984)
  arc A57 (10.260209, 8.249983) -> (9.906656, 8.103537) centre (10.260209, 7.749984) ccw
  line L67 (5.98113, 4.178011) -> (9.906656, 8.103537)
  arc A58 (5.98113, 4.178011) -> (5.834683, 3.824458) centre (6.334682, 3.824458) ccw
  line L68 (5.834683, 0.949998) -> (5.834683, 3.824458)
  line L69 (5.324684, 0) -> (5.834683, 0.949998)
  line L70 (5.834683, -0.949998) -> (5.324684, 0)
  line L71 (5.834683, -3.824458) -> (5.834683, -0.949998)
  arc A59 (5.834683, -3.824458) -> (5.98113, -4.178011) centre (6.334682, -3.824458) ccw
  line L72 (9.906656, -8.103537) -> (5.98113, -4.178011)
  arc A60 (9.906656, -8.103537) -> (10.260209, -8.249984) centre (10.260209, -7.749984) ccw
  line L73 (12.242806, -8.249983) -> (10.260209, -8.249984)
  arc A61 (12.242806, -8.249983) -> (12.7425, -7.732535) centre (12.242806, -7.749984) ccw
  line L74 (12.7425, -4.5625) -> (12.7425, -7.732535)
  arc A62 (13.2425, -4.0625) -> (12.7425, -4.5625) centre (13.2425, -4.5625) ccw
  line L75 (14.49997, -4.0625) -> (13.2425, -4.0625)
  arc A63 (14.99997, -4.5625) -> (14.49997, -4.0625) centre (14.49997, -4.5625) ccw
  line L76 (14.99997, -12.999974) -> (14.99997, -4.5625)
  arc A64 (12.999974, -14.99997) -> (14.99997, -12.999974) centre (12.999974, -12.999974) ccw
  line L77 (4.4375, -14.99997) -> (12.999974, -14.99997)
  arc A65 (3.9375, -14.49997) -> (4.4375, -14.99997) centre (4.4375, -14.49997) ccw
  line L78 (3.9375, -13.2425) -> (3.9375, -14.49997)
  arc A66 (4.4375, -12.7425) -> (3.9375, -13.2425) centre (4.4375, -13.2425) ccw
  line L79 (7.732535, -12.7425) -> (4.4375, -12.7425)
  arc A67 (7.732535, -12.7425) -> (8.249983, -12.242806) centre (7.749985, -12.242806) ccw
  line L80 (8.249984, -10.260209) -> (8.249983, -12.242806)
  arc A68 (8.249984, -10.260209) -> (8.103537, -9.906656) centre (7.749985, -10.260209) ccw
  line L81 (4.178011, -5.98113) -> (8.103537, -9.906656)
  arc A69 (4.178011, -5.98113) -> (3.824458, -5.834683) centre (3.824458, -6.334682) ccw
  line L82 (0.887498, -5.834683) -> (3.824458, -5.834683)
  line L83 (-0.0625, -5.324684) -> (0.887498, -5.834683)
  line L84 (-1.012498, -5.834683) -> (-0.0625, -5.324684)
  line L85 (-3.824458, -5.834683) -> (-1.012498, -5.834683)
  arc A70 (-3.824458, -5.834683) -> (-4.178011, -5.98113) centre (-3.824458, -6.334682) ccw
  line L86 (-8.103537, -9.906656) -> (-4.178011, -5.98113)
  arc A71 (-8.103537, -9.906656) -> (-8.249983, -10.260209) centre (-7.749985, -10.260209) ccw
  line L87 (-8.249984, -12.242806) -> (-8.249983, -10.260209)
  arc A72 (-8.249984, -12.242806) -> (-7.732535, -12.7425) centre (-7.749985, -12.242806) ccw
  line L88 (-4.5625, -12.7425) -> (-7.732535, -12.7425)
  arc A73 (-4.0625, -13.2425) -> (-4.5625, -12.7425) centre (-4.5625, -13.2425) ccw
  line L89 (-4.0625, -14.49997) -> (-4.0625, -13.2425)
  arc A74 (-4.5625, -14.99997) -> (-4.0625, -14.49997) centre (-4.5625, -14.49997) ccw
  line L90 (-12.999974, -14.99997) -> (-4.5625, -14.99997)
  arc A75 (-14.99997, -12.999974) -> (-12.999974, -14.99997) centre (-12.999974, -12.999974) ccw
  line L91 (-14.99997, -4.4375) -> (-14.99997, -12.999974)
  arc A76 (-14.49997, -3.9375) -> (-14.99997, -4.4375) centre (-14.49997, -4.4375) ccw
  line L92 (-13.2425, -3.9375) -> (-14.49997, -3.9375)
  arc A77 (-12.7425, -4.4375) -> (-13.2425, -3.9375) centre (-13.2425, -4.4375) ccw
  line L93 (-12.7425, -7.732535) -> (-12.7425, -4.4375)
  arc A78 (-12.7425, -7.732535) -> (-12.242806, -8.249984) centre (-12.242806, -7.749984) ccw
  line L94 (-10.260209, -8.249983) -> (-12.242806, -8.249984)
  arc A79 (-10.260209, -8.249983) -> (-9.906656, -8.103537) centre (-10.260209, -7.749985) ccw
  line L95 (-5.98113, -4.178011) -> (-9.906656, -8.103537)
  arc A80 (-5.98113, -4.178011) -> (-5.834683, -3.824458) centre (-6.334682, -3.824458) ccw
  line L96 (-5.834683, -0.949998) -> (-5.834683, -3.824458)
  line L97 (-5.324684, 0) -> (-5.834683, -0.949998)
  line L98 (-5.834683, 0.949998) -> (-5.324684, 0)
  line L99 (-5.834683, 3.824458) -> (-5.834683, 0.949998)
  arc A81 (-5.834683, 3.824458) -> (-5.98113, 4.178011) centre (-6.334682, 3.824458) ccw
  line L100 (-9.906656, 8.103537) -> (-5.98113, 4.178011)
  arc A82 (-9.906656, 8.103537) -> (-10.260209, 8.249984) centre (-10.260209, 7.749984) ccw
  line L101 (-12.242806, 8.249983) -> (-10.260209, 8.249984)
  arc A83 (-12.242806, 8.249983) -> (-12.7425, 7.732535) centre (-12.242806, 7.749984) ccw
  line L102 (-12.7425, 4.5625) -> (-12.7425, 7.732535)
  arc A84 (-13.2425, 4.0625) -> (-12.7425, 4.5625) centre (-13.2425, 4.5625) ccw
  line L103 (-14.49997, 4.0625) -> (-13.2425, 4.0625)
  arc A85 (-14.99997, 4.5625) -> (-14.49997, 4.0625) centre (-14.49997, 4.5625) ccw
  line L104 (-14.99997, 25.43744) -> (-14.99997, 4.5625)
  arc A86 (-14.49997, 25.93744) -> (-14.99997, 25.43744) centre (-14.49997, 25.43744) ccw
  line L105 (-13.2425, 25.93744) -> (-14.49997, 25.93744)
  arc A87 (-12.7425, 25.43744) -> (-13.2425, 25.93744) centre (-13.2425, 25.43744) ccw
  arc A88 (-9.499981, -9.87998) -> (-9.87998, -9.499981) centre (-9.87998, -9.87998) ccw
  line L106 (-9.87998, -9.499981) -> (-13.318973, -9.499981)
  arc A89 (-13.318973, -9.499981) -> (-13.699973, -9.88098) centre (-13.318973, -9.88098) ccw
  line L107 (-13.699973, -9.88098) -> (-13.699973, -12.699975)
  arc A90 (-13.699973, -12.699975) -> (-12.699975, -13.699973) centre (-12.699975, -12.699975) ccw
  line L108 (-12.699975, -13.699973) -> (-9.88098, -13.699973)
  arc A91 (-9.88098, -13.699973) -> (-9.499981, -13.318973) centre (-9.88098, -13.318973) ccw
  line L109 (-9.499981, -13.318973) -> (-9.499981, -9.87998)
  arc A92 (12.799974, 19.049962) -> (12.299975, 19.549961) centre (12.299975, 19.049962) ccw
  line L110 (12.299975, 19.549961) -> (9.26818, 19.549961)
  arc A93 (8.207521, 19.9893) -> (9.26818, 19.549961) centre (9.26818, 21.049958) ccw
  line L111 (8.207521, 19.9893) -> (4.178011, 24.01881)
  arc A94 (4.178011, 24.01881) -> (3.824458, 24.165257) centre (3.824458, 23.665258) ccw
  line L112 (3.824458, 24.165257) -> (0.887498, 24.165257)
  line L113 (0.887498, 24.165257) -> (-0.0625, 24.675256)
  line L114 (-0.0625, 24.675256) -> (-1.012498, 24.165257)
  line L115 (-1.012498, 24.165257) -> (-3.824458, 24.165257)
  arc A95 (-3.824458, 24.165257) -> (-4.178011, 24.01881) centre (-3.824458, 23.665258) ccw
  line L116 (-4.178011, 24.01881) -> (-8.207521, 19.9893)
  arc A96 (-9.26818, 19.549961) -> (-8.207521, 19.9893) centre (-9.26818, 21.049958) ccw
  line L117 (-9.26818, 19.549961) -> (-12.299975, 19.549961)
  arc A97 (-12.299975, 19.549961) -> (-12.799974, 19.049962) centre (-12.299975, 19.049962) ccw
  line L118 (-12.799974, 19.049962) -> (-12.799974, 10.949978)
  arc A98 (-12.799974, 10.949978) -> (-12.299975, 10.449979) centre (-12.299975, 10.949978) ccw
  line L119 (-12.299975, 10.449979) -> (-9.26818, 10.449979)
  arc A99 (-8.207521, 10.01064) -> (-9.26818, 10.449979) centre (-9.26818, 8.949982) ccw
  line L120 (-8.207521, 10.01064) -> (-4.178011, 5.98113)
  arc A100 (-4.178011, 5.98113) -> (-3.824458, 5.834683) centre (-3.824458, 6.334682) ccw
  line L121 (-3.824458, 5.834683) -> (-1.012498, 5.834683)
  line L122 (-1.012498, 5.834683) -> (-0.0625, 5.324684)
  line L123 (-0.0625, 5.324684) -> (0.887498, 5.834683)
  line L124 (0.887498, 5.834683) -> (3.824458, 5.834683)
  arc A101 (3.824458, 5.834683) -> (4.178011, 5.98113) centre (3.824458, 6.334682) ccw
  line L125 (4.178011, 5.98113) -> (8.207521, 10.01064)
  arc A102 (9.26818, 10.449979) -> (8.207521, 10.01064) centre (9.26818, 8.949982) ccw
  line L126 (9.26818, 10.449979) -> (12.299975, 10.449979)
  arc A103 (12.299975, 10.449979) -> (12.799974, 10.949978) centre (12.299975, 10.949978) ccw
  line L127 (12.799974, 10.949978) -> (12.799974, 19.049962)
  arc A104 (-9.87998, 39.499921) -> (-9.499981, 39.87992) centre (-9.87998, 39.87992) ccw
  line L128 (-9.499981, 39.87992) -> (-9.499981, 43.318913)
  arc A105 (-9.499981, 43.318913) -> (-9.88098, 43.699913) centre (-9.88098, 43.318913) ccw
  line L129 (-9.88098, 43.699913) -> (-12.699975, 43.699913)
  arc A106 (-12.699975, 43.699913) -> (-13.699973, 42.699915) centre (-12.699975, 42.699915) ccw
  line L130 (-13.699973, 42.699915) -> (-13.699973, 39.88092)
  arc A107 (-13.699973, 39.88092) -> (-13.318973, 39.499921) centre (-13.318973, 39.88092) ccw
  line L131 (-13.318973, 39.499921) -> (-9.87998, 39.499921)
  constraints: 1 other
extrude "Body" add sketch "Sketch" along normal up to surface (150.008319 mm away) from surface at -22.007503
sketch "Sketch2" plane through (0, 0, 0) normal (0, 0, 1) x (1, 0, 0)
  line L0 (0, 0) -> (10, 0)
ref_plane "Work Plane3" through (0, 0, 0) normal (0, -1, 0) x (1, 0, 0)
sketch "Sketch3" plane through (0, 0, 0) normal (0, -1, 0) x (1, 0, 0)
  line L0 (-2, -22.007503) -> (12, -22.007503)
  line L1 (-2, 128.000817) -> (12, 128.000817)
  dimension "d7" = 150.00832
  measures "d7" distance between parallel lines of L0 L1
ref_plane "Work Plane4" through (-12.999978, 1329.99991, 128.000049) normal (0.0003835, 0, 0.9999999) x (0.9999999, 0, -0.0003835)
split "Split1" plane through (-12.999978, 1329.99991, 128.000049) removes the side toward (0.0003835, 0, 0.9999999)
ref_plane "Work Plane5" through (-4.5625, 1329.99991, -22) normal (-0.0003835, 0, -0.9999999) x (-0.9999999, 0, 0.0003835)
split "Split2" plane through (-4.5625, 1329.99991, -22) removes the side toward (-0.0003835, 0, -0.9999999)
equation "\"G_OFFSET_START\" = 22.0075"
equation "\"G_OFFSET_END\" = -14.99917"
equation "\"d2\" = -G_OFFSET_START"
equation "\"d3\" = Length + G_OFFSET_END"
equation "\"G_L\" = d7"
equation "\"Length\" = 142.99999"
body "Solid1"
